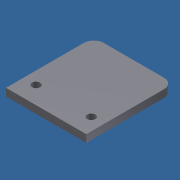
# Autodesk Inventor part: PLACA
Saved by Autodesk Inventor 2012 SP1 (Build 160190100, 190)
## iProperties
Created: 2012-07-23
Part Number: PLACA
Material: Carbon Steel
Document SubType Name: Modeling
Designer: bruno.silveira
Density: 7.87 g/cm^3
Mass: 26.4432 g
Surface Area: 26.42 cm^2
Volume: 3.36 cm^3
Author: bruno.silveira
Autodesk Inventor part; units mm, degrees
ref_plane "YZ Plane" through (0, 0, 0) normal (1, 0, 0) x (0, 1, 0)
ref_plane "XZ Plane" through (0, 0, 0) normal (0, 1, 0) x (-1, 0, 0)
ref_plane "XY Plane" through (0, 0, 0) normal (0, 0, 1) x (1, 0, 0)
sketch "Sketch1" plane through (0, 0, 0) normal (0, 0, 1) x (1, 0, 0)
  line L0 (0, 0) -> (32, 0)
  line L1 (32, 0) -> (32, 35)
  line L2 (32, 35) -> (0, 35)
  line L3 (0, 35) -> (0, 0)
  dimension "d0" = 32
  dimension "d1" = 35
  constraints: 8 end point, 2 parallel, 1 horizontal, 1 perpendicular
  measures "d0" distance of L1.end L2.end
  measures "d1" distance of L2.end L0.start
extrude "Extrusion1" add sketch "Sketch1" along normal blind 3
sketch "Sketch2" plane through (0, 0, 3) normal (0, 0, 1) x (1, 0, 0)
  line L0 (0, 0) -> (0, 35) projected
  line L1 (32, 0) -> (0, 0) projected
  point P0 (5, 7)
  point P1 (27, 7)
  dimension "d4" = 7
  dimension "d5" = 7
  dimension "d6" = 22
  dimension "d7" = 5
  measures "d4" distance from line of L1 point (5, 7)
  measures "d5" distance from line of L1 point (27, 7)
  measures "d6" distance of point (5, 7) point (27, 7)
  measures "d7" distance from line of L0 point (5, 7)
hole "Hole1" at (5, 7, 3) at (27, 7, 3) direction (0, 0, -1) diameter 3.2 depth 8 tip angle 118
fillet "Fillet1" radius 4 2 edges at (32, 35, 1.5) (0, 35, 1.5)
body "Solid1"
